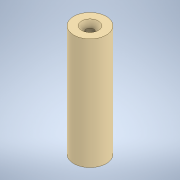
# Autodesk Inventor part: Fuel Grain
Saved by Autodesk Inventor 2021 (Build 250183000, 183)
## iProperties
Created: 2021-02-14
Part Number: Fuel Grain
Material: Acetal Resin, White
Document SubType Name: Modeling
Designer: alexc
Density: 0.932298 g/cm^3
Appearance: Wheat
Mass: 1667.86 g
Surface Area: 1158.06 cm^2
Volume: 1788.98 cm^3
Author: alexc
Autodesk Inventor part; units mm, degrees
ref_plane "YZ Plane" through (0, 0, 0) normal (1, 0, 0) x (0, 1, 0)
ref_plane "XZ Plane" through (0, 0, 0) normal (0, 1, 0) x (-1, 0, 0)
ref_plane "XY Plane" through (0, 0, 0) normal (0, 0, 1) x (1, 0, 0)
sketch "Sketch1" plane through (0, 0, 0) normal (0, 1, 0) x (-1, 0, 0)
  circle A0 centre (0, 0) radius 44.45
  circle A1 centre (0, 0) radius 10
  dimension "d0" = 88.9
  dimension "d1" = 20
  constraints: 2 centre point, 2 coincident
  measures "d0" diameter of A0
  measures "d1" diameter of A1
extrude "Extrusion1" add sketch "Sketch1" along normal blind 304.8
chamfer "Chamfer1" distance 12.7 angle 45 1 edges at (10, 304.8, 0)
equation "\"d2\" = Length"
equation "\"OuterDiameter\" = 127"
equation "\"InnerDiameter\" = 25.4"
equation "\"Length\" = 304.8"
body "Solid1"
